Autodesk Fusion 360 part; units mm, degrees
(part 3 of 3)
sketch "bottom" plane through (23.5, 38.5, -4.6) normal (0, 0, 1) x (1, 0, 0) in component "bottom_shell"
  circle A0 centre (-18.5, 33.5) radius 1.7463 construction
  circle A1 centre (18.5, 33.5) radius 1.7463 construction
  circle A2 centre (18.5, -33.5) radius 1.7463 construction
  circle A3 centre (-18.5, -33.5) radius 1.7463 construction
  line L0 (23.5, -38.5) -> (23.5, 38.5) construction
  line L1 (-23.5, -38.5) -> (23.5, -38.5) construction
  line L2 (-23.5, 38.5) -> (-23.5, -38.5) construction
  line L3 (23.5, 38.5) -> (-23.5, 38.5) construction
  line L4 (25, -39) -> (25, 44.9)
  line L5 (24, 45.9) -> (-24, 45.9)
  line L6 (-25, 44.9) -> (-25, -39)
  line L7 (-24, -40) -> (24, -40)
  arc A4 (25, 44.9) -> (24, 45.9) centre (24, 44.9) ccw
  arc A5 (-24, 45.9) -> (-25, 44.9) centre (-24, 44.9) ccw
  arc A6 (24, -40) -> (25, -39) centre (24, -39) ccw
  arc A7 (-25, -39) -> (-24, -40) centre (-24, -39) ccw
  line L8 (-25.8, 44.9) -> (-25.8, -39)
  arc A8 (-25.8, -39) -> (-24, -40.8) centre (-24, -39) ccw
  line L9 (-24, -40.8) -> (24, -40.8)
  arc A9 (24, -40.8) -> (25.8, -39) centre (24, -39) ccw
  line L10 (25.8, -39) -> (25.8, 44.9)
  arc A10 (25.8, 44.9) -> (24, 46.7) centre (24, 44.9) ccw
  line L11 (24, 46.7) -> (-24, 46.7)
  arc A11 (-24, 46.7) -> (-25.8, 44.9) centre (-24, 44.9) ccw
  line L12 (24, 47.9) -> (-24, 47.9)
  arc A12 (-24, 47.9) -> (-27, 44.9) centre (-24, 44.9) ccw
  line L13 (-27, 44.9) -> (-27, -39)
  arc A13 (-27, -39) -> (-24, -42) centre (-24, -39) ccw
  line L14 (-24, -42) -> (24, -42)
  arc A14 (24, -42) -> (27, -39) centre (24, -39) ccw
  line L15 (27, -39) -> (27, 44.9)
  arc A15 (27, 44.9) -> (24, 47.9) centre (24, 44.9) ccw
  circle A16 centre (-18.5, 33.5) radius 1.75
  circle A17 centre (-18.5, 33.5) radius 3
  circle A18 centre (-18.5, 33.5) radius 5
  circle A19 centre (-18.5, -33.5) radius 1.75
  circle A20 centre (-18.5, -33.5) radius 3
  circle A21 centre (-18.5, -33.5) radius 5
  circle A22 centre (18.5, -33.5) radius 5
  circle A23 centre (18.5, -33.5) radius 3
  circle A24 centre (18.5, -33.5) radius 1.75
  circle A25 centre (18.5, 33.5) radius 1.75
  circle A26 centre (18.5, 33.5) radius 3
  circle A27 centre (18.5, 33.5) radius 5
  line L16 (-20.5, 45.9) -> (-16.5, 45.9)
  line L17 (-16.5, 45.9) -> (-16.5, 39.55)
  line L18 (-17.25, 38.8) -> (-19.75, 38.8)
  line L19 (-20.5, 39.55) -> (-20.5, 45.9)
  line L20 (0, -40) -> (0, 47.9) construction
  arc A28 (-20.5, 39.55) -> (-19.75, 38.8) centre (-19.75, 39.55) ccw
  arc A29 (-17.25, 38.8) -> (-16.5, 39.55) centre (-17.25, 39.55) ccw
  line L21 (-25, 2.95) -> (27, 2.95) construction
  line L22 (-25, 4.95) -> (-24.55, 4.95)
  line L23 (-23.8, 4.2) -> (-23.8, 1.7)
  line L24 (-24.55, 0.95) -> (-25, 0.95)
  line L25 (-25, 0.95) -> (-25, 4.95)
  arc A30 (-23.8, 4.2) -> (-24.55, 4.95) centre (-24.55, 4.2) ccw
  arc A31 (-24.55, 0.95) -> (-23.8, 1.7) centre (-24.55, 1.7) ccw
  line L26 (25, 28.95) -> (24.55, 28.95)
  line L27 (23.8, 28.2) -> (23.8, 25.7)
  line L28 (24.55, 24.95) -> (25, 24.95)
  line L29 (25, 24.95) -> (25, 28.95)
  line L30 (23.5, -38.5) -> (23.5, 38.5)
  arc A32 (24.55, 28.95) -> (23.8, 28.2) centre (24.55, 28.2) ccw
  arc A33 (23.8, 25.7) -> (24.55, 24.95) centre (24.55, 25.7) ccw
  line L31 (25, -23.05) -> (24.55, -23.05)
  arc A34 (23.8, -22.3) -> (24.55, -23.05) centre (24.55, -22.3) ccw
  line L32 (23.8, -22.3) -> (23.8, -19.8)
  arc A35 (24.55, -19.05) -> (23.8, -19.8) centre (24.55, -19.8) ccw
  line L33 (24.55, -19.05) -> (25, -19.05)
  line L34 (-1.25, -38.8) -> (1.25, -38.8)
  line L35 (2, -39.55) -> (2, -40)
  line L36 (2, -40) -> (-2, -40)
  line L37 (-2, -40) -> (-2, -39.55)
  arc A36 (-1.25, -38.8) -> (-2, -39.55) centre (-1.25, -39.55) ccw
  arc A37 (2, -39.55) -> (1.25, -38.8) centre (1.25, -39.55) ccw
  line L38 (11.65, 45.4) -> (-11.65, 45.4) construction
  line L39 (-18.5, 33.5) -> (-18.5, 45.9) construction
  line L40 (16.5, 45.9) -> (16.5, 39.55)
  arc A38 (16.5, 39.55) -> (17.25, 38.8) centre (17.25, 39.55) ccw
  line L41 (17.25, 38.8) -> (19.75, 38.8)
  arc A39 (19.75, 38.8) -> (20.5, 39.55) centre (19.75, 39.55) ccw
  line L42 (20.5, 39.55) -> (20.5, 45.9)
  dimension "d42" = 1
  dimension "d43" = 0.8
  dimension "d44" = 2
  dimension "d48" = 3.5
  dimension "d49" = 6
  dimension "d50" = 10
  dimension "d51" = 3.5
  dimension "d52" = 6
  dimension "d53" = 10
  dimension "d54" = 10
  dimension "d55" = 6
  dimension "d56" = 3.5
  dimension "d57" = 3.5
  dimension "d58" = 6
  dimension "d59" = 10
  dimension "d163" = 1.5
  dimension "d164" = 1.5
  dimension "d165" = 1.5
  dimension "d167" = 4
  dimension "d168" = 0.3
  dimension "d169" = 0.75
  dimension "d170" = 4
  dimension "d171" = 0.3
  dimension "d172" = 0.75
  dimension "d173" = 0.3
  dimension "d174" = 22
  dimension "d175" = 4
  dimension "d176" = 0.75
  dimension "d186" = 4
  dimension "d187" = 0.3
  dimension "d188" = 0.75
  dimension "d231" = 0.5
  constraint parallel L0 L4
  constraint parallel L3 L5
  constraint parallel L2 L6
  constraint parallel L1 L7
  constraint tangent L4 A4
  constraint tangent L5 A4
  constraint tangent L5 A5
  constraint tangent L6 A5
  constraint equal A4 A5
  constraint tangent L4 A6
  constraint tangent L7 A6
  constraint equal A4 A6
  constraint tangent L6 A7
  constraint tangent L7 A7
  constraint equal A4 A7
  constraint concentric A0 A16
  constraint concentric A0 A17
  constraint concentric A17 A18
  constraint concentric A3 A19
  constraint concentric A19 A20
  constraint concentric A19 A21
  constraint concentric A2 A22
  constraint concentric A22 A23
  constraint concentric A23 A24
  constraint concentric A1 A25
  constraint concentric A1 A26
  constraint concentric A25 A27
  constraint horizontal L16
  constraint vertical L17
  constraint horizontal L18
  constraint vertical L19
  constraint coincident L5 L16.start
  constraint midpoint L7 L20.start
  constraint midpoint L12 L20.end
  constraint tangent L18 A28
  constraint tangent L19 A28
  constraint tangent L17 A29
  constraint tangent L18 A29
  constraint equal A28 A29
  constraint midpoint L6 L21.start
  constraint midpoint L15 L21.end
  constraint horizontal L22
  constraint vertical L23
  constraint horizontal L24
  constraint vertical L25
  constraint coincident L6 L22.start
  constraint symmetric L21 L22 L24
  constraint tangent L22 A30
  constraint tangent L23 A30
  constraint tangent L23 A31
  constraint tangent L24 A31
  constraint equal A30 A31
  constraint horizontal L26
  constraint vertical L27
  constraint horizontal L28
  constraint vertical L29
  constraint coincident L4 L26.start
  constraint tangent L26 A32
  constraint tangent L27 A32
  constraint tangent L27 A33
  constraint tangent L28 A33
  constraint equal A32 A33
  constraint symmetric L21 L26.start L31.start
  constraint symmetric L21 L28.end L33.end
  constraint symmetric L21 L26.end L31.end
  constraint symmetric L21 L27.start A34.start
  constraint symmetric L21 A32 A34
  constraint symmetric L21 L27.end L32.end
  constraint symmetric L21 L28.start A35.start
  constraint symmetric L21 A33 A35
  constraint horizontal L34
  constraint vertical L35
  constraint horizontal L36
  constraint vertical L37
  constraint coincident L7 L35.end
  constraint symmetric L20 L35 L37
  constraint tangent L34 A36
  constraint tangent L37 A36
  constraint tangent L34 A37
  constraint tangent L35 A37
  constraint equal A36 A37
  constraint coincident A0.centre A16.centre
  constraint coincident L5 L39.end
  constraint perpendicular L5 L39
  constraint symmetric L17 L19 L39
  constraint symmetric L16.start L20 L42.end
  constraint symmetric L16.end L20 L40.start
  constraint symmetric L20 L18.end L41.end
  constraint symmetric L20 L19.start A39.end
  constraint symmetric L20 A28 A39
  constraint symmetric L20 L17.end L40.end
  constraint symmetric L20 L18.start A38.end
  constraint symmetric L20 A29 A38
  measures "d42" radius of A4
  measures "d48" diameter of A16
  measures "d49" diameter of A17
  measures "d50" diameter of A18
  measures "d51" diameter of A19
  measures "d52" diameter of A20
  measures "d53" diameter of A21
  measures "d54" diameter of A22
  measures "d55" diameter of A23
  measures "d56" diameter of A24
  measures "d57" diameter of A25
  measures "d58" diameter of A26
  measures "d59" diameter of A27
  measures "d163" distance of L1 L7
  measures "d164" distance of L0 L4
  measures "d165" distance of L2 L6
  measures "d167" distance of L17 L19
  measures "d168" distance of L3 L18
  measures "d169" radius of A28
  measures "d170" distance of L22 L24
  measures "d171" distance of L2 L23
  measures "d172" radius of A30
  measures "d173" distance of L27 L30
  measures "d174" distance of L21 L28
  measures "d175" distance of L26 L28
  measures "d176" radius of A32
  measures "d186" distance of L35 L37
  measures "d187" distance of L1 L34
  measures "d188" radius of A36
  measures "d231" distance of L5 L38
extrude "Extrude1'" add sketch "bottom" against normal blind 2 separate body contours L4 L5 L6 L7 A4 A5 A6 A7 L17 L18 L19 A28 A29 L22 L23 L24 A30 A31 L26 L27 L28 A32 A33 L31 A34 L32 A35 L33 L34 L35 L37 A36 A37 L40 A38 L41 A39 L42 | L4 L31 A34 L32 A35 L33 | L7 L34 L35 L36 L37 A36 A37 | L4 L26 L27 L28 L29 A32 A33 | L6 L22 L23 L24 L25 A30 A31 | L5 L40 A38 L41 A39 L42 | L5 L16 L17 L18 L19 A28 A29 | L8 A8 L9 A9 L10 A10 L11 A11 | L12 A12 L13 A13 L14 A14 L15 A15 | A18 | A21 | A22 | A27 makes body 2 in component "bottom_shell"
extrude "Extrude2'" add sketch "bottom" along normal blind 3 contours A17 | A18 | A20 | A21 | A22 | A23 | A26 | A27 bodies 2 in component "bottom_shell"
chamfer "Chamfer1'" distance 2 distance2 2 4 edges at (37.3384, 3.1919, -1.6) (0.3384, 3.1919, -1.6) (0.3384, 70.1919, -1.6) (37.3384, 70.1919, -1.6) measured on face at (45.8915, 4.6647, -1.6) measured on face at (8.8915, 4.6647, -1.6) measured on face at (8.8981, 71.7516, -1.6) measured on face at (45.8981, 71.7516, -1.6) on bodies 2 in component "bottom_shell"
extrude "Extrude3'" add sketch "bottom" along normal blind 11.1 contours L12 A12 L13 A13 L14 A14 L15 A15 bodies 2 in component "bottom_shell"
extrude "Extrude4'" add sketch "bottom" along normal blind 12.6 contours L8 A8 L9 A9 L10 A10 L11 A11 bodies 2 in component "bottom_shell"
fillet "Fillet1" radius 2 8 edges at (23.5, -3.5, -6.6) (-2.6213, -2.6213, -6.6) (-3.5, 41.45, -6.6) (-2.6213, 85.5213, -6.6) (23.5, 86.4, -6.6) (49.6213, 85.5213, -6.6) (50.5, 41.45, -6.6) (49.6213, -2.6213, -6.6) on bodies 2 in component "bottom_shell"
fillet "Fillet2'" radius 0.5 12 edges at (23.5, 84.4, -4.6) (-1.2071, 84.1071, -4.6) (-1.5, 41.45, -4.6) (-1.2071, -1.2071, -4.6) (23.5, -1.5, -4.6) (48.2071, -1.2071, -4.6) (48.5, 41.45, -4.6) (48.2071, 84.1071, -4.6) (37.3384, 73.8081, -4.6) (37.3384, 6.8081, -4.6) (0.3384, 73.8081, -4.6) (0.3384, 6.8081, -4.6) on bodies 2 in component "bottom_shell"
ref_plane "WorkPlane1" through (0, 0, 9) normal (0, 0, 1) x (1, 0, 0) in component "top_shell"
sketch "top" plane through (0, 0, 9) normal (0, 0, 1) x (1, 0, 0) in component "top_shell"
  circle A0 centre (5, 72) radius 1.75 construction
  circle A1 centre (42, 72) radius 1.75 construction
  circle A2 centre (5, 5) radius 1.75 construction
  circle A3 centre (42, 5) radius 1.75 construction
  line L0 (-0.5, -3.5) -> (47.5, -3.5)
  arc A4 (-3.5, -0.5) -> (-0.5, -3.5) centre (-0.5, -0.5) ccw
  line L1 (-3.5, 83.4) -> (-3.5, -0.5)
  arc A5 (47.5, -3.5) -> (50.5, -0.5) centre (47.5, -0.5) ccw
  line L2 (50.5, -0.5) -> (50.5, 83.4)
  line L3 (48.5, -0.5) -> (48.5, 83.4)
  line L4 (-0.5, -1.5) -> (47.5, -1.5)
  arc A6 (47.5, -1.5) -> (48.5, -0.5) centre (47.5, -0.5) ccw
  arc A7 (-1.5, -0.5) -> (-0.5, -1.5) centre (-0.5, -0.5) ccw
  line L5 (-1.5, 83.4) -> (-1.5, -0.5)
  arc A8 (-0.5, 86.4) -> (-3.5, 83.4) centre (-0.5, 83.4) ccw
  arc A9 (-0.5, 84.4) -> (-1.5, 83.4) centre (-0.5, 83.4) ccw
  line L6 (47.5, 84.4) -> (-0.5, 84.4)
  line L7 (47.5, 86.4) -> (-0.5, 86.4)
  arc A10 (48.5, 83.4) -> (47.5, 84.4) centre (47.5, 83.4) ccw
  arc A11 (50.5, 83.4) -> (47.5, 86.4) centre (47.5, 83.4) ccw
  line L8 (10.9538, 9.54) -> (9.525, 9.54) construction
  line L9 (10.9538, 67.96) -> (10.9538, 9.54) construction
  line L10 (9.525, 9.54) -> (8.0963, 9.54) construction
  line L11 (8.0963, 9.54) -> (1.7462, 9.54) construction
  line L12 (1.7462, 9.54) -> (1.7462, 36.6862) construction
  line L13 (1.7462, 36.6862) -> (1.7462, 40.8138) construction
  line L14 (1.7462, 40.8138) -> (1.7462, 62.0863) construction
  line L15 (9.525, 67.96) -> (10.9538, 67.96) construction
  line L16 (8.0963, 67.96) -> (9.525, 67.96) construction
  line L17 (1.7462, 67.96) -> (8.0963, 67.96) construction
  line L18 (1.7462, 63.6738) -> (1.7462, 67.96) construction
  line L19 (30.7975, 15.7163) -> (30.7975, 11.9063) construction
  line L20 (28.8925, 16.3513) -> (30.1625, 16.3513) construction
  line L21 (23.1775, 11.2713) -> (25.0825, 11.2713) construction
  line L22 (23.1775, 11.9063) -> (23.1775, 15.7163) construction
  line L23 (23.1775, 11.9063) -> (23.1775, 11.2713) construction
  line L24 (23.8125, 16.3513) -> (25.0825, 16.3513) construction
  line L25 (28.8925, 11.2713) -> (30.1625, 11.2713) construction
  circle A12 centre (23, 65) radius 1.4 construction
  line L26 (35.3458, 34.4408) -> (46.2518, 34.4408)
  line L27 (46.2518, 34.4408) -> (46.2518, 21.7568)
  line L28 (46.2518, 21.7568) -> (35.3458, 21.7568)
  line L29 (35.3458, 21.7568) -> (35.3458, 34.4408)
  line L30 (11.4538, 68.46) -> (1.2462, 68.46)
  line L31 (1.2462, 68.46) -> (1.2462, 9.04)
  line L32 (1.2462, 9.04) -> (11.4538, 9.04)
  line L33 (11.4538, 9.04) -> (11.4538, 68.46)
  circle A13 centre (23, 65) radius 2
  circle A14 centre (40, 56.5) radius 2
  line L34 (47.5, 85.6) -> (-0.5, 85.6)
  arc A15 (-0.5, 85.6) -> (-2.7, 83.4) centre (-0.5, 83.4) ccw
  line L35 (-2.7, 83.4) -> (-2.7, -0.5)
  arc A16 (-2.7, -0.5) -> (-0.5, -2.7) centre (-0.5, -0.5) ccw
  line L36 (-0.5, -2.7) -> (47.5, -2.7)
  arc A17 (47.5, -2.7) -> (49.7, -0.5) centre (47.5, -0.5) ccw
  line L37 (49.7, -0.5) -> (49.7, 83.4)
  arc A18 (49.7, 83.4) -> (47.5, 85.6) centre (47.5, 83.4) ccw
  circle A19 centre (5, 72) radius 1.25
  circle A20 centre (5, 72) radius 3
  circle A21 centre (42, 72) radius 1.25
  circle A22 centre (42, 72) radius 3
  circle A23 centre (42, 5) radius 1.25
  circle A24 centre (42, 5) radius 3
  circle A25 centre (5, 5) radius 1.25
  circle A26 centre (5, 5) radius 3
  line L38 (28.6703, 53.848) -> (15.4623, 53.848) construction
  line L39 (15.4623, 18.542) -> (15.4623, 53.848) construction
  line L40 (28.6703, 18.542) -> (28.6703, 53.848) construction
  line L41 (15.4623, 18.542) -> (20.7963, 18.542) construction
  line L42 (23.3362, 18.542) -> (28.6703, 18.542) construction
  line L43 (35.687, 9.398) -> (16.383, 9.398) construction
  line L44 (16.383, 9.398) -> (16.383, 7.366) construction
  arc A27 (23.3363, 18.542) -> (20.7963, 18.542) centre (22.0663, 18.542) ccw construction
  arc A28 (16.383, 5.334) -> (16.383, 7.366) centre (16.383, 6.35) ccw construction
  line L45 (16.383, 3.302) -> (16.383, 5.334) construction
  line L46 (16.383, 3.302) -> (35.687, 3.302) construction
  line L47 (35.687, 9.398) -> (35.687, 3.302) construction
  line L48 (15.4623, 54.348) -> (28.6703, 54.348)
  line L49 (29.1703, 53.848) -> (29.1703, 18.542)
  line L50 (28.6703, 18.042) -> (15.4623, 18.042)
  line L51 (14.9623, 18.542) -> (14.9623, 53.848)
  line L52 (16.383, 9.898) -> (35.687, 9.898)
  line L53 (36.187, 9.398) -> (36.187, 3.302)
  line L54 (35.687, 2.802) -> (16.383, 2.802)
  line L55 (15.883, 3.302) -> (15.883, 9.398)
  arc A29 (15.4623, 54.348) -> (14.9623, 53.848) centre (15.4623, 53.848) ccw
  arc A30 (29.1703, 53.848) -> (28.6703, 54.348) centre (28.6703, 53.848) ccw
  arc A31 (28.6703, 18.042) -> (29.1703, 18.542) centre (28.6703, 18.542) ccw
  arc A32 (14.9623, 18.542) -> (15.4623, 18.042) centre (15.4623, 18.542) ccw
  arc A33 (15.883, 3.302) -> (16.383, 2.802) centre (16.383, 3.302) ccw
  arc A34 (16.383, 9.898) -> (15.883, 9.398) centre (16.383, 9.398) ccw
  arc A35 (36.187, 9.398) -> (35.687, 9.898) centre (35.687, 9.398) ccw
  arc A36 (35.687, 2.802) -> (36.187, 3.302) centre (35.687, 3.302) ccw
  circle A37 centre (40, 56.5) radius 1.5
  line L56 (39.1478, 33.9408) -> (35.8458, 33.9408) construction
  line L57 (42.4498, 33.9408) -> (39.1478, 33.9408) construction
  line L58 (45.7518, 33.9408) -> (42.4498, 33.9408) construction
  line L59 (45.7518, 22.2568) -> (45.7518, 33.9408) construction
  line L60 (42.4498, 22.2568) -> (45.7518, 22.2568) construction
  line L61 (39.1478, 22.2568) -> (42.4498, 22.2568) construction
  line L62 (35.8458, 22.2568) -> (39.1478, 22.2568) construction
  line L63 (35.8458, 33.9408) -> (35.8458, 22.2568) construction
  line L64 (35.5, 15.6) -> (36.7, 15.6) construction
  line L65 (36.7, 15.6) -> (38.3, 15.6) construction
  line L66 (38.3, 15.6) -> (39.2, 15.6) construction
  line L67 (39.2, 15.6) -> (40.8, 15.6) construction
  line L68 (40.8, 15.6) -> (41.7, 15.6) construction
  line L69 (41.7, 15.6) -> (43.3, 15.6) construction
  line L70 (44.6, 15.6) -> (43.3, 15.6) construction
  line L71 (44.6, 12) -> (44.6, 15.6) construction
  line L72 (44.6, 12) -> (43.3, 12) construction
  line L73 (41.7, 12) -> (43.3, 12) construction
  line L74 (40.8, 12) -> (41.7, 12) construction
  line L75 (39.2, 12) -> (40.8, 12) construction
  line L76 (38.3, 12) -> (39.2, 12) construction
  line L77 (36.7, 12) -> (38.3, 12) construction
  line L78 (35.5, 12) -> (36.7, 12) construction
  line L79 (35.5, 15.6) -> (35.5, 12) construction
  line L80 (35.4, 53.3) -> (36.7, 53.3) construction
  line L81 (38.3, 53.3) -> (36.7, 53.3) construction
  line L82 (39.2, 53.3) -> (38.3, 53.3) construction
  line L83 (40.8, 53.3) -> (39.2, 53.3) construction
  line L84 (41.7, 53.3) -> (40.8, 53.3) construction
  line L85 (43.3, 53.3) -> (41.7, 53.3) construction
  line L86 (44.5, 53.3) -> (43.3, 53.3) construction
  line L87 (44.5, 49.7) -> (44.5, 53.3) construction
  line L88 (44.5, 49.7) -> (43.3, 49.7) construction
  line L89 (43.3, 49.7) -> (41.7, 49.7) construction
  line L90 (41.7, 49.7) -> (40.8, 49.7) construction
  line L91 (40.8, 49.7) -> (39.2, 49.7) construction
  line L92 (39.2, 49.7) -> (38.3, 49.7) construction
  line L93 (38.3, 49.7) -> (36.7, 49.7) construction
  line L94 (35.4, 49.7) -> (36.7, 49.7) construction
  line L95 (35.4, 53.3) -> (35.4, 49.7) construction
  line L96 (34.9, 53.8) -> (45, 53.8)
  line L97 (45, 53.8) -> (45, 49.2)
  line L98 (45, 49.2) -> (34.9, 49.2)
  line L99 (34.9, 49.2) -> (34.9, 53.8)
  line L100 (35, 16.1) -> (45.1, 16.1)
  line L101 (45.1, 16.1) -> (45.1, 11.5)
  line L102 (45.1, 11.5) -> (35, 11.5)
  line L103 (35, 11.5) -> (35, 16.1)
  line L104 (35.8458, 35.9408) -> (45.7518, 35.9408)
  line L105 (47.7518, 33.9408) -> (47.7518, 22.2568)
  line L106 (45.7518, 20.2568) -> (35.8458, 20.2568)
  line L107 (33.8458, 22.2568) -> (33.8458, 33.9408)
  arc A38 (35.8458, 35.9408) -> (33.8458, 33.9408) centre (35.8458, 33.9408) ccw
  arc A39 (33.8458, 22.2568) -> (35.8458, 20.2568) centre (35.8458, 22.2568) ccw
  arc A40 (45.7518, 20.2568) -> (47.7518, 22.2568) centre (45.7518, 22.2568) ccw
  arc A41 (47.7518, 33.9408) -> (45.7518, 35.9408) centre (45.7518, 33.9408) ccw
  line L108 (34.8, 17.3) -> (45.3, 17.3)
  line L109 (46.3, 16.3) -> (46.3, 11.3)
  line L110 (45.3, 10.3) -> (34.8, 10.3)
  line L111 (33.8, 11.3) -> (33.8, 16.3)
  arc A42 (34.8, 17.3) -> (33.8, 16.3) centre (34.8, 16.3) ccw
  arc A43 (46.3, 16.3) -> (45.3, 17.3) centre (45.3, 16.3) ccw
  arc A44 (45.3, 10.3) -> (46.3, 11.3) centre (45.3, 11.3) ccw
  arc A45 (33.8, 11.3) -> (34.8, 10.3) centre (34.8, 11.3) ccw
  point P0 (47.5, -0.5)
  dimension "d90" = 0.5
  dimension "d91" = 0.5
  dimension "d92" = 0.5
  dimension "d93" = 0.5
  dimension "d94" = 4
  dimension "d95" = 4
  dimension "d96" = 1.2
  dimension "d99" = 2.5
  dimension "d100" = 6
  dimension "d101" = 2.5
  dimension "d102" = 6
  dimension "d103" = 2.5
  dimension "d104" = 6
  dimension "d105" = 2.5
  dimension "d106" = 6
  dimension "d117" = 0.5
  dimension "d118" = 0.5
  dimension "d119" = 0.5
  dimension "d120" = 0.5
  dimension "d121" = 0.5
  dimension "d122" = 0.5
  dimension "d123" = 0.5
  dimension "d124" = 0.5
  dimension "d125" = 0.5
  dimension "d137" = 0.5
  dimension "d138" = 0.5
  dimension "d139" = 0.5
  dimension "d140" = 0.5
  dimension "d141" = 0.5
  dimension "d142" = 0.5
  dimension "d143" = 0.5
  dimension "d144" = 0.5
  dimension "d145" = 0.5
  dimension "d146" = 0.5
  dimension "d147" = 0.5
  dimension "d148" = 0.5
  dimension "d189" = 1.5
  dimension "d190" = 1.5
  dimension "d191" = 1.5
  dimension "d192" = 1.5
  dimension "d193" = 2
  dimension "d194" = 2
  dimension "d195" = 1.2
  dimension "d196" = 1.2
  dimension "d197" = 1.2
  dimension "d198" = 1.2
  dimension "d199" = 1
  constraint horizontal L26
  constraint vertical L27
  constraint horizontal L28
  constraint vertical L29
  constraint horizontal L30
  constraint vertical L31
  constraint horizontal L32
  constraint vertical L33
  constraint concentric A12 A13
  constraint concentric A0 A19
  constraint concentric A0 A20
  constraint concentric A1 A21
  constraint concentric A1 A22
  constraint concentric A3 A23
  constraint concentric A23 A24
  constraint concentric A2 A25
  constraint concentric A2 A26
  constraint horizontal L48
  constraint vertical L49
  constraint horizontal L50
  constraint vertical L51
  constraint horizontal L52
  constraint vertical L53
  constraint horizontal L54
  constraint vertical L55
  constraint tangent L48 A29
  constraint tangent L51 A29
  constraint tangent L48 A30
  constraint tangent L49 A30
  constraint equal A29 A30
  constraint tangent L49 A31
  constraint tangent L50 A31
  constraint equal A29 A31
  constraint tangent L50 A32
  constraint tangent L51 A32
  constraint equal A29 A32
  constraint tangent L54 A33
  constraint tangent L55 A33
  constraint equal A29 A33
  constraint tangent L52 A34
  constraint tangent L55 A34
  constraint equal A29 A34
  constraint tangent L52 A35
  constraint tangent L53 A35
  constraint equal A29 A35
  constraint tangent L53 A36
  constraint tangent L54 A36
  constraint equal A29 A36
  constraint concentric A14 A37
  constraint horizontal L96
  constraint vertical L97
  constraint horizontal L98
  constraint vertical L99
  constraint horizontal L100
  constraint vertical L101
  constraint horizontal L102
  constraint vertical L103
  constraint horizontal L104
  constraint vertical L105
  constraint horizontal L106
  constraint vertical L107
  constraint tangent L104 A38
  constraint tangent L107 A38
  constraint tangent L106 A39
  constraint tangent L107 A39
  constraint tangent L105 A40
  constraint tangent L106 A40
  constraint equal A39 A40
  constraint tangent L104 A41
  constraint tangent L105 A41
  constraint equal A39 A41
  constraint horizontal L108
  constraint vertical L109
  constraint horizontal L110
  constraint vertical L111
  constraint tangent L108 A42
  constraint tangent L111 A42
  constraint tangent L108 A43
  constraint tangent L109 A43
  constraint equal A42 A43
  constraint tangent L109 A44
  constraint tangent L110 A44
  constraint equal A42 A44
  constraint tangent L110 A45
  constraint tangent L111 A45
  constraint equal A42 A45
  measures "d90" distance of L9 L33
  measures "d91" distance of L12 L31
  measures "d92" distance of L11 L32
  measures "d93" distance of L17 L30
  measures "d94" diameter of A13
  measures "d95" diameter of A14
  measures "d99" diameter of A19
  measures "d100" diameter of A20
  measures "d101" diameter of A21
  measures "d102" diameter of A22
  measures "d103" diameter of A23
  measures "d104" diameter of A24
  measures "d105" diameter of A25
  measures "d106" diameter of A26
  measures "d117" distance of L38 L48
  measures "d118" distance of L40 L49
  measures "d119" distance of L39 L51
  measures "d120" distance of L41 L50
  measures "d121" distance of L43 L52
  measures "d122" distance of L46 L54
  measures "d123" distance of L45 L55
  measures "d124" distance of L47 L53
  measures "d125" radius of A29
  measures "d137" distance of L26 L56
  measures "d138" distance of L29 L63
  measures "d139" distance of L28 L62
  measures "d140" distance of L27 L59
  measures "d141" distance of L79 L103
  measures "d142" distance of L71 L101
  measures "d143" distance of L65 L100
  measures "d144" distance of L77 L102
  measures "d145" distance of L80 L96
  measures "d146" distance of L94 L98
  measures "d147" distance of L95 L99
  measures "d148" distance of L87 L97
  measures "d189" distance of L26 L104
  measures "d190" distance of L28 L106
  measures "d191" distance of L29 L107
  measures "d192" distance of L27 L105
  measures "d193" radius of A38
  measures "d194" radius of A39
  measures "d195" distance of L102 L110
  measures "d196" distance of L100 L108
  measures "d197" distance of L101 L109
  measures "d198" distance of L103 L111
  measures "d199" radius of A42
extrude "Extrude1''" add sketch "top" along normal blind 2 separate body contours L0 A4 L1 A5 L2 A8 L7 A11 | L3 L4 A6 A7 L5 A9 L6 A10 | L34 A15 L35 A16 L36 A17 L37 A18 | A19 | A20 | A21 | A22 | A23 | A24 | A25 | A26 | L48 L49 L50 L51 A29 A30 A31 A32 | L52 L53 L54 L55 A33 A34 A35 A36 | L96 L97 L98 L99 | L104 L105 L106 L107 A38 A39 A40 A41 | L108 L109 L110 L111 A42 A43 A44 A45 makes body 3 in component "top_shell"
extrude "Extrude2''" add sketch "top" against normal blind 2.5 contours L0 A4 L1 A5 L2 A8 L7 A11 bodies 3 in component "top_shell"
extrude "Extrude3''" add sketch "top" against normal blind 1 contours L34 A15 L35 A16 L36 A17 L37 A18 bodies 3 in component "top_shell"
extrude "Extrude4''" add sketch "top" against normal blind 9 contours A20 | A22 | A24 | A26 bodies 3 in component "top_shell"
fillet "Fillet1'" radius 2 8 edges at (23.5, 86.4, 11) (-2.6213, 85.5213, 11) (-3.5, 41.45, 11) (-2.6213, -2.6213, 11) (23.5, -3.5, 11) (49.6213, -2.6213, 11) (50.5, 41.45, 11) (49.6213, 85.5213, 11) on bodies 3 in component "top_shell"
extrude "Extrude5'" cut sketch "top" along normal blind 1 contours L48 L49 L50 L51 A29 A30 A31 A32 | L52 L53 L54 L55 A33 A34 A35 A36 bodies 3 in component "top_shell"
extrude "Extrude7" add sketch "top" against normal blind 3 contours L104 L105 L106 L107 A38 A39 A40 A41 bodies 3 in component "top_shell"
extrude "Extrude8'" add sketch "top" against normal blind 4.5 contours L108 L109 L110 L111 A42 A43 A44 A45 bodies 3 in component "top_shell"
fillet "Fillet2''" radius 0.5 8 edges at (35, 11.5, 10) (35, 16.1, 10) (45.1, 16.1, 10) (45.1, 11.5, 10) (35.3458, 34.4408, 10) (35.3458, 21.7568, 10) (46.2518, 21.7568, 10) (46.2518, 34.4408, 10) on bodies 3 in component "top_shell"
extrude "Extrude7'" add sketch "bottom" along normal blind 4.6 contours L4 L31 A34 L32 A35 L33 | L7 L34 L35 L36 L37 A36 A37 | L4 L26 L27 L28 L29 A32 A33 | L6 L22 L23 L24 L25 A30 A31 | L5 L40 A38 L41 A39 L42 | L5 L16 L17 L18 L19 A28 A29 bodies 2 in component "bottom_shell"
sketch "switch (2)" plane through (0, 86.4, 0) normal (0, 1, 0) x (-1, 0, 0) in component "bottom_shell"
  line L0 (-47.5, -4.6) -> (0.5, -4.6)
  line L1 (0.5, -4.6) -> (0.5, 6.5)
  line L2 (0.5, 6.5) -> (-47.5, 6.5)
  line L3 (-47.5, 6.5) -> (-47.5, -4.6)
  line L4 (-28.2, -2.5) -> (-28.2, 1.8) construction
  line L5 (-18.8, -2.5) -> (-28.2, -2.5) construction
  line L6 (-18.8, 1.8) -> (-18.8, -2.5) construction
  line L7 (-28.2, 1.8) -> (-18.8, 1.8) construction
  line L8 (-29.2, 2.5) -> (-17.8, 2.5)
  line L9 (-17.8, 2.5) -> (-17.8, -3.2)
  line L10 (-17.8, -3.2) -> (-29.2, -3.2)
  line L11 (-29.2, -3.2) -> (-29.2, 2.5)
  dimension "d233" = 0.7
  dimension "d234" = 0.7
  dimension "d235" = 1
  dimension "d236" = 1
  constraint horizontal L8
  constraint vertical L9
  constraint horizontal L10
  constraint vertical L11
  measures "d233" distance of L7 L8
  measures "d234" distance of L5 L10
  measures "d235" distance of L6 L9
  measures "d236" distance of L4 L11
extrude "Extrude9'" cut sketch "switch (2)" against normal blind 2 contours L8 L9 L10 L11 bodies 2 in component "bottom_shell"
fillet "Fillet3" radius 0.5 4 edges at (29.2, 85.4, 2.5) (17.8, 85.4, 2.5) (17.8, 85.4, -3.2) (29.2, 85.4, -3.2) on bodies 2 in component "bottom_shell"
fillet "Fillet3'" radius 0.5 16 edges at (35.4922, 34.2944, 11) (35.3458, 28.0988, 11) (35.4922, 21.9032, 11) (40.7988, 21.7568, 11) (46.1054, 21.9032, 11) (46.2518, 28.0988, 11) (46.1054, 34.2944, 11) (40.7988, 34.4408, 11) (35.1464, 15.9536, 11) (35, 13.8, 11) (35.1464, 11.6464, 11) (40.05, 11.5, 11) (44.9536, 11.6464, 11) (45.1, 13.8, 11) (44.9536, 15.9536, 11) (40.05, 16.1, 11) on bodies 3 in component "top_shell"
fillet "Fillet4" radius 0.5 4 edges at (1.2462, 9.04, 10) (11.4538, 9.04, 10) (11.4538, 68.46, 10) (1.2462, 68.46, 10) on bodies 3 in component "top_shell"
chamfer "Chamfer1''" distance 0.5 angle 45 8 edges at (1.2462, 38.75, 11) (1.3926, 68.3136, 11) (6.35, 68.46, 11) (11.3074, 68.3136, 11) (11.4538, 38.75, 11) (11.3074, 9.1864, 11) (6.35, 9.04, 11) (1.3926, 9.1864, 11) on bodies 3 in component "top_shell"
chamfer "Chamfer2" distance 0.5 angle 45 2 edges at (21.1353, 65.7232, 11) (38.1353, 57.2232, 11) on bodies 3 in component "top_shell"
sketch "Label" plane through (0, 0, 11) normal (0, 0, 1) x (-1, 0, 0) in component "Label"
  circle A0 centre (-23, -65) radius 2.5 construction
  arc A1 (-35.5, -16.6) -> (-34.5, -15.6) centre (-35.5, -15.6) ccw construction
  line L0 (-35.5, -16.6) -> (-44.6, -16.6) construction
  arc A2 (-45.6, -15.6) -> (-44.6, -16.6) centre (-44.6, -15.6) ccw construction
  line L1 (-45.6, -15.6) -> (-45.6, -12) construction
  arc A3 (-44.6, -11) -> (-45.6, -12) centre (-44.6, -12) ccw construction
  line L2 (-44.6, -11) -> (-35.5, -11) construction
  arc A4 (-34.5, -12) -> (-35.5, -11) centre (-35.5, -12) ccw construction
  line L3 (-34.5, -12) -> (-34.5, -15.6) construction
  line L4 (-47.5, -84.4) -> (0.5, -84.4)
  arc A5 (0.5, -84.4) -> (1.5, -83.4) centre (0.5, -83.4) ccw
  line L5 (1.5, -83.4) -> (1.5, 0.5)
  arc A6 (1.5, 0.5) -> (0.5, 1.5) centre (0.5, 0.5) ccw
  line L6 (0.5, 1.5) -> (-47.5, 1.5)
  arc A7 (-47.5, 1.5) -> (-48.5, 0.5) centre (-47.5, 0.5) ccw
  line L7 (-48.5, 0.5) -> (-48.5, -83.4)
  arc A8 (-48.5, -83.4) -> (-47.5, -84.4) centre (-47.5, -83.4) ccw
  arc A9 (-35.8458, -34.9408) -> (-34.8458, -33.9408) centre (-35.8458, -33.9408) ccw construction
  line L8 (-35.8458, -34.9408) -> (-45.7518, -34.9408) construction
  arc A10 (-46.7518, -33.9408) -> (-45.7518, -34.9408) centre (-45.7518, -33.9408) ccw construction
  line L9 (-46.7518, -33.9408) -> (-46.7518, -22.2568) construction
  arc A11 (-45.7518, -21.2568) -> (-46.7518, -22.2568) centre (-45.7518, -22.2568) ccw construction
  line L10 (-45.7518, -21.2568) -> (-35.8458, -21.2568) construction
  arc A12 (-34.8458, -22.2568) -> (-35.8458, -21.2568) centre (-35.8458, -22.2568) ccw construction
  line L11 (-34.8458, -22.2568) -> (-34.8458, -33.9408) construction
  line L12 (-0.7462, -9.54) -> (-0.7462, -67.96) construction
  arc A13 (-1.7462, -68.96) -> (-0.7462, -67.96) centre (-1.7462, -67.96) ccw construction
  line L13 (-1.7462, -68.96) -> (-10.9538, -68.96) construction
  arc A14 (-11.9538, -67.96) -> (-10.9538, -68.96) centre (-10.9538, -67.96) ccw construction
  line L14 (-11.9538, -67.96) -> (-11.9538, -9.54) construction
  arc A15 (-10.9538, -8.54) -> (-11.9538, -9.54) centre (-10.9538, -9.54) ccw construction
  line L15 (-10.9538, -8.54) -> (-1.7462, -8.54) construction
  arc A16 (-0.7462, -9.54) -> (-1.7462, -8.54) centre (-1.7462, -9.54) ccw construction
  circle A17 centre (-40, -56.5) radius 2.5 construction
  line L16 (-0.2462, -9.54) -> (-0.2462, -67.96)
  arc A18 (-1.7462, -69.46) -> (-0.2462, -67.96) centre (-1.7462, -67.96) ccw
  line L17 (-1.7462, -69.46) -> (-10.9538, -69.46)
  arc A19 (-12.4538, -67.96) -> (-10.9538, -69.46) centre (-10.9538, -67.96) ccw
  line L18 (-12.4538, -67.96) -> (-12.4538, -9.54)
  arc A20 (-10.9538, -8.04) -> (-12.4538, -9.54) centre (-10.9538, -9.54) ccw
  line L19 (-10.9538, -8.04) -> (-1.7462, -8.04)
  arc A21 (-0.2462, -9.54) -> (-1.7462, -8.04) centre (-1.7462, -9.54) ccw
  line L20 (-44.6, -10.5) -> (-35.5, -10.5)
  arc A22 (-34, -12) -> (-35.5, -10.5) centre (-35.5, -12) ccw
  line L21 (-34, -12) -> (-34, -15.6)
  arc A23 (-35.5, -17.1) -> (-34, -15.6) centre (-35.5, -15.6) ccw
  line L22 (-35.5, -17.1) -> (-44.6, -17.1)
  arc A24 (-46.1, -15.6) -> (-44.6, -17.1) centre (-44.6, -15.6) ccw
  line L23 (-46.1, -15.6) -> (-46.1, -12)
  arc A25 (-44.6, -10.5) -> (-46.1, -12) centre (-44.6, -12) ccw
  line L24 (-45.7518, -20.7568) -> (-35.8458, -20.7568)
  arc A26 (-34.3458, -22.2568) -> (-35.8458, -20.7568) centre (-35.8458, -22.2568) ccw
  line L25 (-34.3458, -22.2568) -> (-34.3458, -33.9408)
  arc A27 (-35.8458, -35.4408) -> (-34.3458, -33.9408) centre (-35.8458, -33.9408) ccw
  line L26 (-35.8458, -35.4408) -> (-45.7518, -35.4408)
  arc A28 (-47.2518, -33.9408) -> (-45.7518, -35.4408) centre (-45.7518, -33.9408) ccw
  line L27 (-47.2518, -33.9408) -> (-47.2518, -22.2568)
  arc A29 (-45.7518, -20.7568) -> (-47.2518, -22.2568) centre (-45.7518, -22.2568) ccw
  circle A30 centre (-23, -65) radius 3
  circle A31 centre (-40, -56.5) radius 3
  line L28 (-23.5, -81.8) -> (-24.9142, -83.2142)
  line L29 (-24.9142, -83.2142) -> (-23.5, -84.4)
  line L30 (-23.5, -84.4) -> (-22.0858, -83.2142)
  line L31 (-22.0858, -83.2142) -> (-23.5, -81.8)
  line L32 (-11.85, -83.9) -> (-11.85, -83.5) construction
  line L33 (-35.15, -83.5) -> (-35.15, -83.9) construction
  line L34 (-35.15, -83.5) -> (-11.85, -83.5) construction
  line L35 (-23.5, -81.8) -> (-23.5, -84.4) construction
  dimension "d210" = 0.5
  dimension "d211" = 0.5
  dimension "d212" = 0.5
  dimension "d213" = 0.5
  dimension "d214" = 0.5
  dimension "d217" = 2
  dimension "d218" = 2
  constraint coincident L33.start L34.start
  constraint coincident L32.end L34.end
  constraint perpendicular L4 L35
  constraint symmetric L33.start L32.end L35
  constraint coincident L4 L29.end
  measures "d217" distance of L28.start L28.end
  measures "d218" distance of L28.start L30.end
extrude "Extrude1'''" add sketch "Label" along normal blind 0.2 separate body contours L28 L29 L30 L31 | L4 A5 L5 A6 L6 A7 L7 A8 makes body 4 in component "Label"
component "PCB" placed x (1, 0, 0) y (0, 1, 0) z (0, 0, 1) at (0, 0, 0)
component "bottom_shell" placed x (1, 0, 0) y (0, 1, 0) z (0, 0, 1) at (0, 0, 0)
component "top_shell" placed x (1, 0, 0) y (0, 1, 0) z (0, 0, 1) at (0, 0, 0)
component "Label" placed x (1, 0, 0) y (0, 1, 0) z (0, 0, 1) at (0, 0, 0)
equation "wall = 2 mm"
equation "below = 3 mm"
equation "above = 9 mm"
equation "wall_distance = 1.5 mm"
equation "d39 = -below - 1.6 mm"
equation "inner_radius = 1 mm"
equation "d42 = inner_radius"
equation "d43 = wall * 0.4"
equation "d44 = wall"
equation "bottom_drill = 3.5 mm"
equation "bottom_screw = 6 mm"
equation "bottom_post = 10 mm"
equation "d48 = bottom_drill"
equation "d49 = bottom_screw"
equation "d50 = bottom_post"
equation "d51 = bottom_drill"
equation "d52 = bottom_screw"
equation "d53 = bottom_post"
equation "d54 = bottom_post"
equation "d55 = bottom_screw"
equation "d56 = bottom_drill"
equation "d57 = bottom_drill"
equation "d58 = bottom_screw"
equation "d59 = bottom_post"
equation "d60 = -wall"
equation "d62 = below"
equation "overlap = 1.5 mm"
equation "top_height = wall + overlap + 1 mm"
equation "pcb = 1.6 mm"
equation "total_height = above + pcb + below + 2 * wall"
equation "bottom_height = total_height - top_height"
equation "d71 = bottom_height - wall"
equation "d73 = bottom_height - wall + overlap"
equation "fillet = 2 mm"
equation "d77 = fillet"
equation "d80 = above"
equation "cutout_distance = 0.5 mm"
equation "d90 = cutout_distance"
equation "d91 = cutout_distance"
equation "d92 = cutout_distance"
equation "d93 = cutout_distance"
equation "d95 = d94"
equation "d96 = wall * 0.6"
equation "top_post = 6 mm"
equation "top_drill = 2.5 mm"
equation "d99 = top_drill"
equation "d100 = top_post"
equation "d101 = top_drill"
equation "d102 = top_post"
equation "d103 = top_drill"
equation "d104 = top_post"
equation "d105 = top_drill"
equation "d106 = top_post"
equation "d107 = wall"
equation "d109 = -top_height + wall"
equation "d111 = -top_height + wall + overlap"
equation "d113 = -above"
equation "d116 = fillet"
equation "d117 = cutout_distance"
equation "d118 = cutout_distance"
equation "d119 = cutout_distance"
equation "d120 = cutout_distance"
equation "d121 = cutout_distance"
equation "d122 = cutout_distance"
equation "d123 = cutout_distance"
equation "d124 = cutout_distance"
equation "d125 = cutout_distance"
equation "ic_indent = 1 mm"
equation "d127 = ic_indent"
equation "d137 = cutout_distance"
equation "d138 = cutout_distance"
equation "d139 = cutout_distance"
equation "d140 = cutout_distance"
equation "d141 = cutout_distance"
equation "d142 = cutout_distance"
equation "d143 = cutout_distance"
equation "d144 = cutout_distance"
equation "d145 = cutout_distance"
equation "d146 = cutout_distance"
equation "d147 = cutout_distance"
equation "d148 = cutout_distance"
equation "d163 = wall_distance"
equation "d164 = wall_distance"
equation "d165 = wall_distance"
equation "tol = 0.3 mm"
equation "d168 = tol"
equation "d170 = d167"
equation "d171 = tol"
equation "d172 = d169"
equation "d173 = tol"
equation "d175 = d167"
equation "d177 = below + pcb"
equation "d186 = d170"
equation "d187 = tol"
equation "d190 = d189"
equation "d191 = d189"
equation "d192 = d189"
equation "d196 = d195"
equation "d197 = d195"
equation "d198 = d195"
equation "d234 = d233"
equation "d236 = d235"
equation "d237 = -wall"
named bodies: "pcb", "bottom_shell", "top_shell"
